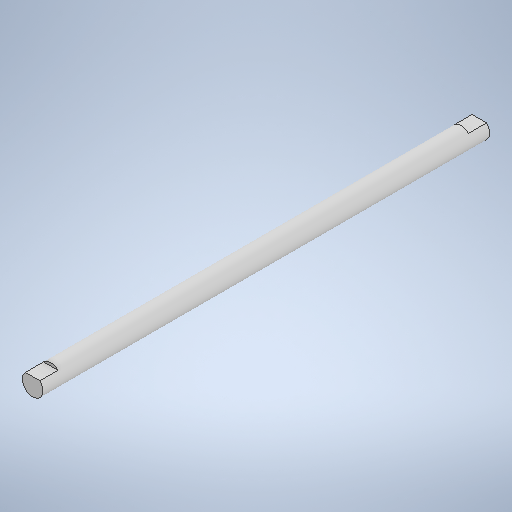
# Autodesk Inventor part: Project_stationary_rod
Saved by Autodesk Inventor 2025 (Build 290162000, 162)
## iProperties
Created: 2025-08-31
Part Number: Project_stationary_rod
Material: Generic
Document SubType Name: Modeling
Designer: Kiran
Density: 1 g/cm^3
Appearance: Default
Author: Kiran
Autodesk Inventor part; units mm, degrees
ref_plane "YZ Plane" through (0, 0, 0) normal (1, 0, 0) x (0, 1, 0)
ref_plane "XZ Plane" through (0, 0, 0) normal (0, 1, 0) x (-1, 0, 0)
ref_plane "XY Plane" through (0, 0, 0) normal (0, 0, 1) x (1, 0, 0)
sketch "Sketch2" plane through (0, 0, 0) normal (0, 0, 1) x (1, 0, 0)
  circle A0 centre (0, 0) radius 8.5
  dimension "d4" = 17
  constraints: 1 centre point, 1 coincident
  measures "d4" diameter of A0
extrude "Extrusion2" add sketch "Sketch2" along normal blind 370
sketch "Sketch3" plane through (0, 0, 370) normal (0, 0, 1) x (1, 0, 0)
  circle A0 centre (0, 0) radius 8.5 projected
  arc A1 (6.0104, 6.0104) -> (-6.0104, 6.0104) centre (0, 0) ccw
  line L0 (0, 0) -> (6.0104, 6.0104) construction
  line L1 (0, 0) -> (8.5, 0) construction
  line L2 (0, 0) -> (-6.0104, 6.0104) construction
  arc A2 (6.0104, 6.0104) -> (-6.0104, 6.0104) centre (0, 0) ccw
  line L3 (6.0104, 6.0104) -> (-6.0104, 6.0104)
  point P0 (-6.0104, 6.0104)
  dimension "d7" = 45
  constraints: 8 end point, 4 point on circle, 2 centre point, 2 horizontal, 1 coincident, 1 concentric, 1 equal length, 2 other
  measures "d7" angle of L1 L0
extrude "Extrusion3" cut sketch "Sketch3" against normal blind 15 contours L3 A0 picked at (-0.3172, 6.8225)
sketch "Sketch4" plane through (0, 0, 0) normal (0, 0, -1) x (-1, 0, 0)
  arc A0 (-6.0104, 6.0104) -> (6.0104, 6.0104) centre (0, 0) ccw projected
  arc A1 (6.0104, 6.0104) -> (-6.0104, 6.0104) centre (0, 0) ccw
  line L0 (0, 0) -> (-6.0104, 6.0104) construction
  line L1 (0, 0) -> (6.0104, 6.0104) construction
  arc A2 (-6.0104, 6.0104) -> (6.0104, 6.0104) centre (0, 12.0208) ccw
  line L2 (-6.0104, 6.0104) -> (6.0104, 6.0104) projected
  line L3 (-6.0104, 6.0104) -> (6.0104, 6.0104)
  dimension "d11" = 90
  constraints: 6 end point, 5 point on circle, 2 centre point, 2 tangent, 1 coincident
  measures "d11" angle of L1 L0
extrude "Extrusion4" cut sketch "Sketch4" against normal blind 15 contours A1 L2
body "Solid2"
